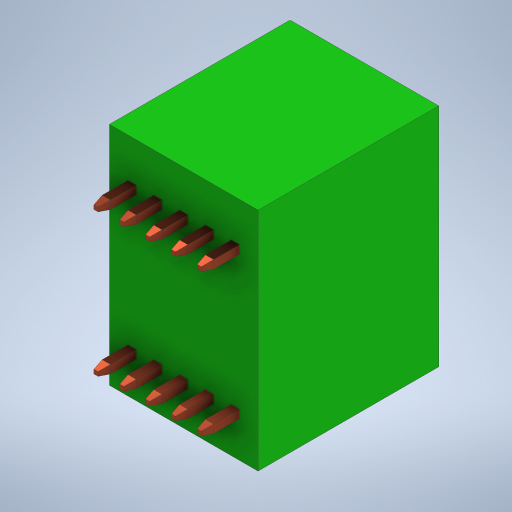
# Autodesk Inventor part: DB2EVH-2.5-2-5P-GN
Saved by Autodesk Inventor 2024 (Build 280153000, 153)
## iProperties
Created: 2023-05-23
Part Number: DB2EVH-2.5-2-5P-GN
Material: Generic
Document SubType Name: Modeling
Designer: torba
Density: 1 g/cm^3
Appearance: Default
Author: torba
Autodesk Inventor part; units mm, degrees
ref_plane "YZ Plane" through (0, 0, 0) normal (1, 0, 0) x (0, 1, 0)
ref_plane "XZ Plane" through (0, 0, 0) normal (0, 1, 0) x (-1, 0, 0)
ref_plane "XY Plane" through (0, 0, 0) normal (0, 0, 1) x (1, 0, 0)
sketch "Sketch1" plane through (0, 0, 0) normal (0, 0, 1) x (1, 0, 0)
  line L0 (0, 0) -> (14.4, 0)
  line L1 (14.4, 0) -> (14.4, -21.9)
  line L2 (14.4, -21.9) -> (0, -21.9)
  line L3 (0, -21.9) -> (0, 0)
  line L4 (1.8, -18.4) -> (2.6, -18.4)
  line L5 (2.6, -18.4) -> (2.6, -17.6)
  line L6 (2.6, -17.6) -> (1.8, -17.6)
  line L7 (1.8, -17.6) -> (1.8, -18.4)
  line L8 (1.8, -18.4) -> (2.6, -17.6) construction
  point P0 (2.2, -18)
  dimension "d0" = 14.4
  dimension "d1" = 21.9
  dimension "d2" = 0.8
  dimension "d3" = 0.8
  dimension "d5" = 3.9
  dimension "d6" = 2.2
  dimension "d14" = 0
  dimension "d15" = 0
  dimension "d22" = 12.2
  constraints: 18 end point, 4 parallel, 2 horizontal, 2 perpendicular, 1 midpoint
  measures "d0" distance between parallel lines of L1 L3
  measures "d1" distance between parallel lines of L2 L0
  measures "d2" distance of L4.end L5.end
  measures "d3" distance of L4.start L4.end
  measures "d5" distance from line of L2 point (2.2, -18)
  measures "d6" distance from line of L3 point (2.2, -18)
  measures "d14" distance from line of point (0, 0) L3
  measures "d15" distance from line of point (0, 0) L0
  measures "d22" distance from line of point (2.2, -18) L1
extrude "Extrusion1" add sketch "Sketch1" along normal blind 3.5 and the other way blind 17.5 contours L7 L6 L5 L4
chamfer "Chamfer1" distance 0.2 distance2 1 4 edges at (2.6, -18, 3.5) (2.2, -18.4, 3.5) (1.8, -18, 3.5) (2.2, -17.6, 3.5) measured on face at (2.3333, -18.1333, 3.5)
chamfer "Chamfer2" distance 0.2 distance2 1 4 edges at (1.8, -18, -17.5) (2.2, -17.6, -17.5) (2.6, -18, -17.5) (2.2, -18.4, -17.5) measured on face at (2.3333, -18.1333, -17.5)
extrude "Extrusion2" add sketch "Sketch1" against normal blind 17.5 separate body contours L0 L1 L2 L3 | L7 L6 L5 L4
pattern_linear "Rectangular Pattern1" count 2 spacing 13.8 along (0, 1, 0) count 5 spacing 2.5 along (1, 0, 0) of "Extrusion1", "Chamfer1", "Chamfer2" bodies 1
sketch "Sketch2" plane through (0, 0, -17.5) normal (0, 0, -1) x (-1, 0, 0)
  point P0 (0, 0)
sketch "Sketch3" plane through (0, 0, -17.5) normal (0, 0, -1) x (-1, 0, 0)
  line L0 (-1.8, -17.6) -> (-1.8, -18.4) projected
  line L1 (-1.8, -18.4) -> (-1.8, -17.6) projected
  line L2 (-2.6, -18.4) -> (-2.6, -17.6) projected
  line L3 (-2.6, -17.6) -> (-2.6, -18.4) projected
  line L4 (-1.8, -17.6) -> (-2.6, -17.6) projected
  line L5 (-1.8, -18.4) -> (-2.6, -18.4) projected
  line L6 (-2.6, -18.4) -> (-1.8, -18.4) projected
  line L7 (-2.6, -17.6) -> (-1.8, -17.6) projected
  line L8 (-1.8, -17.6) -> (-2.6, -17.6) projected
  line L9 (-0.6, -15.8) -> (-0.6, -21.4)
  line L10 (-0.6, -21.4) -> (-2.37, -21.4)
  line L11 (-2.37, -21.4) -> (-2.37, -20.15)
  line L12 (-2.37, -20.15) -> (-10.59, -20.15)
  line L13 (-10.59, -20.15) -> (-10.59, -21.4)
  line L14 (-10.59, -21.4) -> (-12.36, -21.4)
  line L15 (-12.36, -21.4) -> (-12.36, -20.15)
  line L16 (-12.36, -20.15) -> (-13.8, -20.15)
  line L17 (-13.8, -20.15) -> (-13.8, -15.8)
  line L18 (-13.8, -15.8) -> (-0.6, -15.8)
  line L19 (0, -21.9) -> (0, 0) projected
  line L20 (-14.4, 0) -> (-14.4, -21.9) projected
  line L21 (-14.4, -21.9) -> (0, -21.9) projected
  point P0 (-2.2, -18.4)
  point P1 (-12.36, -20.775)
  dimension "d23" = 14.4
  dimension "d25" = 1.77
  dimension "d26" = 1.77
  dimension "d27" = 2.2
  dimension "d28" = 1.44
  dimension "d29" = 0.6
  dimension "d31" = 0.6
  dimension "d32" = 0.5
  dimension "d33" = 5.6
  dimension "d34" = 1.25
  constraints: 20 end point, 7 perpendicular, 4 point on line, 2 midpoint, 1 vertical
  measures "d23" distance between parallel lines of L19 L20
  measures "d25" distance between parallel lines of L11 L9
  measures "d26" distance between parallel lines of L13 L15
  measures "d27" distance from line of L19 point (-2.2, -18.4)
  measures "d28" distance from line of L17 point (-12.36, -20.775)
  measures "d29" distance between parallel lines of L20 L17
  measures "d31" distance between parallel lines of L9 L19
  measures "d32" distance between parallel lines of L21 L10
  measures "d33" distance between parallel lines of L10 L18
  measures "d34" distance between parallel lines of L10 L12
extrude "Extrusion3" cut sketch "Sketch3" against normal blind 10 contours L0 L5 L2 L4 | L9 L10 L11 L12 L13 L14 L15 L16 L17 L18 bodies 2
pattern_linear "Rectangular Pattern2" count 2 spacing 13.8 along (0, 1, 0) of "Extrusion3" bodies 2
equation "\"d3\" = d2"
equation "\"d25\" = d26"
body "Solid1"
